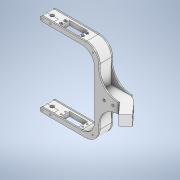
# Autodesk Inventor part: Soporte
Saved by Autodesk Inventor 2022 (Build 260153000, 153)
## iProperties
Created: 2021-10-11
Part Number: Soporte
Material: Aluminum 6061-AHC
Document SubType Name: Modeling
Designer: juanp
Density: 2.7 g/cm^3
Appearance: Aluminum - Dark
Author: juanp
Autodesk Inventor part; units mm, degrees
sketch "Sketch1" plane through (0, 0, 0) normal (0, 1, 0) x (-1, 0, 0)
  line L0 (-19.95, 9.85) -> (19.95, 9.85) construction
  line L1 (19.95, 9.85) -> (19.95, -9.85) construction
  line L2 (19.95, -9.85) -> (-19.95, -9.85) construction
  line L3 (-19.95, -9.85) -> (-19.95, 9.85) construction
  line L4 (-19.95, 9.85) -> (19.95, -9.85) construction
  line L5 (19.95, 9.85) -> (-19.95, -9.85) construction
  line L6 (19.95, 0) -> (24.7111, 0) construction
  line L7 (-19.95, 0) -> (-24.7111, 0) construction
  line L8 (24.7111, 4.925) -> (24.7111, -4.925) construction
  line L9 (-24.7111, 4.925) -> (-24.7111, -4.925) construction
  circle A0 centre (24.7111, 4.925) radius 1.65
  circle A1 centre (24.7111, -4.925) radius 1.65
  circle A2 centre (-24.7111, 4.925) radius 1.65
  circle A3 centre (-24.7111, -4.925) radius 1.65
  line L10 (20.45, 10.35) -> (-20.45, 10.35)
  line L11 (-20.45, 10.35) -> (-20.45, -10.35)
  line L12 (-20.45, -10.35) -> (20.45, -10.35)
  line L13 (20.45, -10.35) -> (20.45, 10.35)
  line L14 (20.45, 10.35) -> (-20.45, -10.35) construction
  line L15 (-20.45, 10.35) -> (20.45, -10.35) construction
  line L16 (19.95, 0) -> (-10.1, 0) construction
  circle A4 centre (-10.1, 0) radius 1.5 construction
  line L17 (-10.1, 0) -> (49.9, 0) construction
  circle A5 centre (49.9, 0) radius 4
  line L18 (63.9, 10.35) -> (-69.6, 10.35)
  line L19 (-69.6, 10.35) -> (-69.6, -15.05)
  line L20 (-69.6, -15.05) -> (63.9, -15.05)
  line L21 (-59.6, 10.35) -> (-59.6, -15.05)
  line L22 (63.9, 10.35) -> (63.9, -15.05)
  line L23 (45.9, 0) -> (35.9, 0)
  line L24 (35.9, 0) -> (35.9, 10.35)
  line L25 (53.9, 0) -> (63.9, 0)
  point P0 (0, 0)
  point P1 (20.25, -10.15)
  point P2 (-20.25, -10.15)
  point P3 (45.0352, 10.15)
  point P4 (53.0352, 10.15)
  dimension "d0" = 39.9
  dimension "d1" = 19.7
  dimension "d2" = 4.7611
  dimension "d3" = 3.3
  dimension "d4" = 9.85
  dimension "d5" = 0.5
  dimension "d6" = 0.5
  dimension "d7" = 30.05
  dimension "d8" = 3
  dimension "d9" = 60
  dimension "d12" = 8
  dimension "d44" = 119.5
  dimension "d46" = 0
  dimension "d48" = 10
  dimension "d89" = 4.7
  dimension "d93" = 10
  dimension "d94" = 10
  dimension "d99" = 25.4
  constraints: 52 end point, 8 midpoint, 8 point on line, 7 horizontal, 6 centre point, 6 coincident, 4 parallel, 4 perpendicular, 4 vertical, 3 equal radius, 2 equal length, 2 point on circle
  measures "d0" distance between parallel lines of L1 L3
  measures "d1" distance between parallel lines of L2 L0
  measures "d2" distance of L6.end L6.start
  measures "d3" diameter of A0
  measures "d4" distance of L8.start L8.end
  measures "d5" distance between parallel lines of L3 L11
  measures "d6" distance between parallel lines of L2 L12
  measures "d7" distance of L6.start L16.end
  measures "d8" diameter of A4
  measures "d9" distance of L17.start L17.end
  measures "d12" diameter of A5
  measures "d44" distance from line of L19 A5.centre
  measures "d46" distance between parallel lines of L18 L10
  measures "d48" distance between parallel lines of L19 L21
  measures "d89" distance between parallel lines of L12 L20
  measures "d93" distance edge to line of A5 L22
  measures "d94" distance of L23.start L23.end
  measures "d99" distance between parallel lines of L18 L20
extrude "Extrusion1" add sketch "Sketch1" along normal blind 10 contours L18 L24 L23 A5 L25 L22 L20 L21 L11 L12 L13 | L21 L20 L19 L18
extrude "Extrusion18" add sketch "Sketch1" along normal up to surface (10 mm away) separate body contours L18 L22 L25 A5 L23 L24
ref_plane "Work Plane1" through (0, 94.85, 0) normal (0, 1, 0) x (1, 0, 0)
sketch "Sketch10" plane through (0, 0, 0) normal (0, -1, 0) x (1, 0, 0)
  circle A0 centre (-24.7111, 4.925) radius 1.65 projected
  circle A1 centre (-24.7111, -4.925) radius 1.65 projected
  circle A2 centre (24.7111, -4.925) radius 1.65 projected
  circle A3 centre (24.7111, 4.925) radius 1.65 projected
  line L0 (-26.3075, 7.69) -> (-23.1148, 7.69)
  line L1 (-23.1148, 7.69) -> (-21.5184, 4.925)
  line L2 (-21.5184, 4.925) -> (-23.1148, 2.16)
  line L3 (-23.1148, 2.16) -> (-26.3075, 2.16)
  line L4 (-26.3075, 2.16) -> (-27.9039, 4.925)
  line L5 (-27.9039, 4.925) -> (-26.3075, 7.69)
  line L6 (-26.3075, -7.69) -> (-27.9039, -4.925)
  line L7 (-27.9039, -4.925) -> (-26.3075, -2.16)
  line L8 (-26.3075, -2.16) -> (-23.1148, -2.16)
  line L9 (-23.1148, -2.16) -> (-21.5184, -4.925)
  line L10 (-21.5184, -4.925) -> (-23.1148, -7.69)
  line L11 (-23.1148, -7.69) -> (-26.3075, -7.69)
  line L12 (26.3075, -7.69) -> (23.1148, -7.69)
  line L13 (23.1148, -7.69) -> (21.5184, -4.925)
  line L14 (21.5184, -4.925) -> (23.1148, -2.16)
  line L15 (23.1148, -2.16) -> (26.3075, -2.16)
  line L16 (26.3075, -2.16) -> (27.9039, -4.925)
  line L17 (27.9039, -4.925) -> (26.3075, -7.69)
  line L18 (27.9039, 4.925) -> (26.3075, 2.16)
  line L19 (26.3075, 2.16) -> (23.1148, 2.16)
  line L20 (23.1148, 2.16) -> (21.5184, 4.925)
  line L21 (21.5184, 4.925) -> (23.1148, 7.69)
  line L22 (23.1148, 7.69) -> (26.3075, 7.69)
  line L23 (26.3075, 7.69) -> (27.9039, 4.925)
  point P0 (0, 0)
  dimension "d66" = 5.53
  constraints: 48 end point, 4 coincident, 4 horizontal, 3 equal length, 52 other
  measures "d66" distance between parallel lines of L21 L18
extrude "Extrusion11" cut sketch "Sketch10" against normal blind 2.3 contours A0 | A1 | A2 | A3 | L0 L1 L2 L3 L4 L5 | L6 L7 L8 L9 L10 L11 | L12 L13 L14 L15 L16 L17 | L18 L19 L20 L21 L22 L23 bodies 1
mirror "Mirror1" about plane through (0, 94.85, 0) normal (0, 1, 0) of "Extrusion1", "Extrusion11" bodies 1
extrude "Extrusion7" add sketch "Sketch1" along normal up to surface (179.7 mm away) contours L21 L20 L19 L18 bodies 1
fillet "Fillet4" radius 30 4 edges at (59.6, 179.7, -2.35) (69.6, 189.7, -2.35) (59.6, 10, -2.35) (69.6, 0, -2.35)
mirror "Mirror3" about plane through (0, 94.85, 0) normal (0, 1, 0) of "Extrusion18" bodies 2
sketch "Sketch15" plane through (-63.9, 0, 10.35) normal (0, 0, 1) x (1, 0, 0)
  line L0 (18, 10) -> (28, 10) projected
  line L1 (0, 10) -> (10, 10) projected
  line L2 (10, 10) -> (18, 10) construction
  line L3 (18, 0) -> (28, 0) projected
  line L4 (18, 10) -> (28, 0) construction
  line L5 (10, 10) -> (0, 0) construction
  circle A0 centre (23, 5) radius 1.65
  circle A1 centre (5, 5) radius 1.65
  line L6 (18, 179.7) -> (28, 179.7) projected
  line L7 (0, 179.7) -> (10, 179.7) projected
  line L8 (10, 179.7) -> (18, 179.7) construction
  line L9 (18, 179.7) -> (28, 189.7) construction
  line L10 (10, 179.7) -> (0, 189.7) construction
  circle A2 centre (23, 184.7) radius 1.65
  circle A3 centre (5, 184.7) radius 1.65
  line L11 (114.7132, 18.7868) -> (124.7132, 8.7868) construction
  arc A4 (103.5, 0) -> (133.5, 30) centre (103.5, 30) ccw projected
  arc A5 (93.5, 10) -> (123.5, 40) centre (93.5, 40) ccw projected
  arc A6 (123.5, 149.7) -> (93.5, 179.7) centre (93.5, 149.7) ccw projected
  arc A7 (133.5, 159.7) -> (103.5, 189.7) centre (103.5, 159.7) ccw projected
  line L12 (124.7132, 180.9132) -> (114.7132, 170.9132) construction
  circle A8 centre (119.7132, 13.7868) radius 1.65
  circle A9 centre (119.7132, 175.9132) radius 1.65
  point P0 (63.9, 0)
  dimension "d97" = 3.3
  dimension "d98" = 3.3
  dimension "d102" = 3.3
  dimension "d103" = 3.3
  dimension "d104" = 3.3
  dimension "d105" = 3.3
  constraints: 12 end point, 6 centre point, 6 midpoint, 4 line through centre, 4 point on circle, 1 coincident
  measures "d97" diameter of A0
  measures "d98" diameter of A1
  measures "d102" diameter of A2
  measures "d103" diameter of A3
  measures "d104" diameter of A8
  measures "d105" diameter of A9
extrude "Extrusion19" cut sketch "Sketch15" against normal through all bodies 2 1
ref_plane "Work Plane4" through (-63.9, 0, -2.35) normal (0, 0, -1) x (-1, 0, 0)
sketch "Sketch17" plane through (-63.9, 0, -15.05) normal (0, 0, -1) x (-1, 0, 0)
  circle A0 centre (-23, 184.7) radius 1.65 projected
  circle A1 centre (-5, 5) radius 1.65 projected
  circle A2 centre (-119.7132, 175.9132) radius 1.65 projected
  circle A3 centre (-5, 184.7) radius 1.65 projected
  circle A4 centre (-23, 5) radius 1.65 projected
  circle A5 centre (-119.7132, 13.7868) radius 1.65 projected
  arc A6 (-133.5, 30) -> (-103.5, 0) centre (-103.5, 30) ccw projected
  line L0 (-103.5, 0) -> (0, 0) projected
  line L1 (0, 0) -> (0, 10) projected
  line L2 (-93.5, 10) -> (0, 10) projected
  arc A7 (-123.5, 40) -> (-93.5, 10) centre (-93.5, 40) ccw projected
  line L3 (-123.5, 40) -> (-123.5, 149.7) projected
  arc A8 (-93.5, 179.7) -> (-123.5, 149.7) centre (-93.5, 149.7) ccw projected
  line L4 (-93.5, 179.7) -> (0, 179.7) projected
  line L5 (0, 189.7) -> (0, 179.7) projected
  line L6 (-103.5, 189.7) -> (0, 189.7) projected
  arc A9 (-103.5, 189.7) -> (-133.5, 159.7) centre (-103.5, 159.7) ccw projected
  line L7 (-133.5, 159.7) -> (-133.5, 30) projected
  line L8 (-178, 106.05) -> (-133.5, 106.05)
  line L9 (-133.5, 106.05) -> (-133.5, 83.65)
  line L10 (-133.5, 83.65) -> (-178, 83.65)
  line L11 (-178, 83.65) -> (-178, 106.05)
  line L12 (-133.5, 159.7) -> (-133.5, 30) projected
  arc A10 (-178, 106.05) -> (-133.5, 150.55) centre (-178, 150.55) ccw
  arc A11 (-133.5, 39.15) -> (-178, 83.65) centre (-178, 39.15) ccw
  line L13 (-133.5, 159.7) -> (-133.5, 30) projected
  line L14 (-10, 179.7) -> (-18, 179.7) projected
  line L15 (-10, 189.7) -> (-10, 179.7) construction
  line L16 (-18, 189.7) -> (-10, 189.7) projected
  line L17 (-18, 189.7) -> (-18, 179.7) construction
  line L18 (-10, 10) -> (-18, 10) projected
  line L19 (-18, 0) -> (-18, 10) construction
  line L20 (-18, 0) -> (-10, 0) projected
  line L21 (-10, 0) -> (-10, 10) construction
  line L22 (-18, 179.7) -> (-10, 179.7) projected
  line L23 (-14, 179.7) -> (-14, 10) construction
  point P0 (-63.9, 0)
  point P1 (-133.5, 94.85)
  point P2 (-133.5, 39.15)
  dimension "d113" = 22.4
  dimension "d114" = 164
  constraints: 10 end point, 4 midpoint, 4 point on circle, 4 tangent, 3 point on line, 2 centre point, 2 parallel, 1 equal radius, 1 horizontal, 1 perpendicular
  measures "d113" distance between parallel lines of L8 L10
  measures "d114" distance between parallel lines of L11 L23
extrude "Extrusion21" add sketch "Sketch17" along normal blind 3 separate body
mirror "Mirror4" about plane through (-63.9, 0, -2.35) normal (0, 0, -1) of "Extrusion21" bodies 3
sketch "Sketch19" plane through (69.6, 30, -15.05) normal (1, 0, 0) x (0, 0, -1)
  line L0 (-25.4, 53.65) -> (-28.4, 53.65) projected
  line L1 (0, 76.05) -> (3, 76.05) projected
  line L2 (-25.4, 53.65) -> (0, 53.65)
  line L3 (0, 53.65) -> (0, 76.05)
  line L4 (0, 76.05) -> (-25.4, 76.05)
  line L5 (-25.4, 76.05) -> (-25.4, 53.65)
  point P0 (-15.05, -30)
  constraints: 8 end point, 2 parallel, 1 horizontal, 1 perpendicular
extrude "Extrusion23" add sketch "Sketch19" along normal up to surface (44.5 mm away) separate body
ref_plane "Work Plane5" through (114.1, 106.05, 10.35) normal (0.6755902, 0, 0.7372773) x (0, -1, 0)
sketch "Sketch20" plane through (114.1, 106.05, 10.35) normal (0.6755902, 0, 0.7372773) x (0, -1, 0)
  line L0 (0, 0) -> (22.4, 0) projected
  line L1 (22.4, 0) -> (0, 0) projected
  line L2 (22.4, 0) -> (0, 0)
  line L3 (0, 0) -> (0, 22.4)
  line L4 (0, 22.4) -> (22.4, 22.4)
  line L5 (22.4, 22.4) -> (22.4, 0)
  point P0 (106.05, -77.131)
  constraints: 8 end point, 2 parallel, 2 perpendicular, 1 horizontal
extrude "Extrusion24" add sketch "Sketch20" along normal blind 35 bodies 4
sketch "Sketch21" plane through (69.6, 83.65, -15.05) normal (0, -1, 0) x (1, 0, 0)
  line L0 (44.5, 25.4) -> (44.5, 0) projected
  line L1 (44.5, 0) -> (0, 0) projected
  arc A0 (44.5, 0) -> (61.015, 10.2668) centre (34.4117, 34.6442) ccw
  line L2 (61.015, 10.2668) -> (84.6607, 36.0715) projected
  line L3 (44.5, 25.4) -> (61.015, 10.2668) projected
  point P0 (-69.6, 15.05)
  constraints: 2 point on circle, 1 centre point, 1 tangent
extrude "Extrusion25" add sketch "Sketch21" against normal up to surface (22.4 mm away) bodies 4
fillet "Fillet6" radius 3 16 edges at (-63.9, 189.7, -7.525) (-63.9, 179.7, -7.525) (-63.9, 10, -7.525) (-63.9, 0, -7.525) (-63.9, 189.7, 5.175) (-63.9, 179.7, 5.175) (-63.9, 10, 5.175) (-63.9, 0, 5.175) (-63.9, 189.7, 11.85) (-63.9, 189.7, -16.55) (-63.9, 179.7, 11.85) (-63.9, 179.7, -16.55) (-63.9, 10, 11.85) (-63.9, 0, 11.85) (-63.9, 0, -16.55) (-63.9, 10, -16.55)
sketch "Sketch22" plane through (-63.9, 0, -18.05) normal (0, 0, -1) x (-1, 0, 0)
  line L0 (-133.5, 83.65) -> (-133.5, 106.05) construction
  line L1 (-178, 83.65) -> (-178, 106.05) construction
  line L2 (-133.5, 94.85) -> (-145.75, 94.85) construction
  line L3 (-145.75, 94.85) -> (-165.75, 94.85) construction
  line L4 (-165.75, 94.85) -> (-178, 94.85) construction
  circle A0 centre (-145.75, 94.85) radius 2.65
  circle A1 centre (-165.75, 94.85) radius 2.65
  point P0 (-63.9, 0)
  dimension "d123" = 20
  dimension "d124" = 5.3
  dimension "d125" = 5.3
  constraints: 6 end point, 2 centre point, 2 coincident, 2 midpoint, 1 collinear, 1 horizontal, 1 point on line
  measures "d123" distance of L2.end L3.end
  measures "d124" diameter of A0
  measures "d125" diameter of A1
extrude "Extrusion26" cut sketch "Sketch22" against normal through all bodies 3 4
sketch "Sketch23" plane through (114.1, 83.65, 10.35) normal (-0.7372773, 0, 0.6755902) x (0.6755902, 0, 0.7372773)
  line L0 (0, 0) -> (0, 22.4) projected
  line L1 (0, 0) -> (35, 0) projected
  line L2 (35, 22.4) -> (35, 0) projected
  line L3 (0, 22.4) -> (35, 22.4) projected
  line L4 (0, 22.4) -> (35, 22.4) projected
  line L5 (-1, 22.4) -> (-1, 0) construction
  line L6 (0, 0) -> (35, 0) projected
  line L7 (35, 22.4) -> (35, 0) projected
  line L8 (35, 11.2) -> (24.5, 11.2) construction
  line L9 (24.5, 11.2) -> (9.5, 11.2) construction
  line L10 (9.5, 11.2) -> (-1, 11.2) construction
  circle A0 centre (24.5, 11.2) radius 2.65
  circle A1 centre (9.5, 11.2) radius 2.65
  point P0 (-84.7157, -83.65)
  dimension "d129" = 15
  dimension "d130" = 5.3
  dimension "d133" = 10.5
  dimension "d134" = 1
  constraints: 8 end point, 3 point on line, 2 centre point, 2 coincident, 2 midpoint, 1 collinear, 1 equal radius, 1 horizontal, 1 perpendicular
  measures "d129" distance of L8.end L9.end
  measures "d130" diameter of A0
  measures "d133" distance of L9.end L10.end
  measures "d134" distance between parallel lines of L0 L5
extrude "Extrusion27" cut sketch "Sketch23" against normal through all contours A0 | A1 bodies 4
ref_plane "Work Plane3" through (0, 94.85, 0) normal (0, 1, 0) x (1, 0, 0)
body "Solid1"
body "Solid3"
body "Solid4"
body "Solid5"
